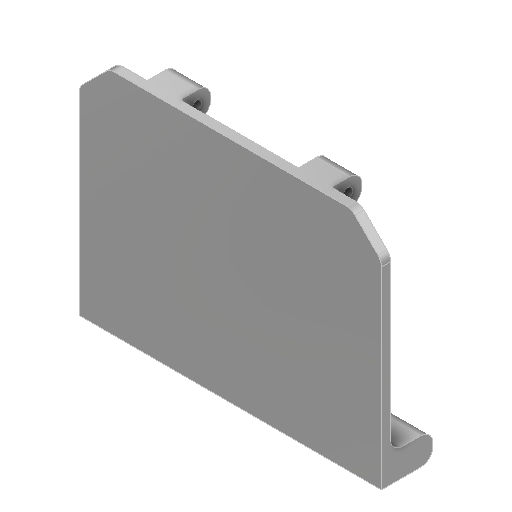
# Autodesk Inventor part: 3DP_PLA_Stand_Leg
Saved by Autodesk Inventor 2026.1 (Build 301233000, 233)
## iProperties
Created: 2024-09-01
Part Number: 3DP_PLA_Stand_Leg
Material: Generic
Document SubType Name: Modeling
Designer: User
Density: 1 g/cm^3
Appearance: Rubber - Black - Version 1.1
Author: User
Autodesk Inventor part; units mm, degrees
ref_plane "YZ Plane" through (0, 0, 0) normal (1, 0, 0) x (0, 1, 0)
ref_plane "XZ Plane" through (0, 0, 0) normal (0, 1, 0) x (-1, 0, 0)
ref_plane "XY Plane" through (0, 0, 0) normal (0, 0, 1) x (1, 0, 0)
sketch "Sketch1" plane through (0, 0, 0) normal (0, 0, 1) x (1, 0, 0)
  line L0 (-30.5, 4.5) -> (-19.5, 4.5)
  line L1 (-19.5, 4.5) -> (-19.5, -4.5)
  line L2 (-19.5, -4.5) -> (-30.5, -4.5)
  line L3 (-30.5, -4.5) -> (-30.5, 4.5)
  line L4 (19.5, 4.5) -> (30.5, 4.5)
  line L5 (30.5, 4.5) -> (30.5, -4.5)
  line L6 (30.5, -4.5) -> (19.5, -4.5)
  line L7 (19.5, -4.5) -> (19.5, 4.5)
  line L8 (-50, 4.5) -> (50, 4.5)
  line L9 (50, 4.5) -> (50, -71)
  line L10 (50, -71) -> (-50, -71)
  line L11 (-50, -71) -> (-50, 4.5)
  point P0 (0, 0)
  dimension "d0" = 11
  dimension "d1" = 9
  dimension "d2" = 19.5
  dimension "d3" = 4.5
  dimension "d4" = 11
  dimension "d5" = 19.5
  dimension "d6" = 9
  dimension "d7" = 100
  dimension "d8" = 50
  dimension "d9" = 4.5
  dimension "d10" = 71
  constraints: 24 end point, 6 parallel, 3 horizontal, 3 perpendicular
  measures "d0" distance of L1.end L2.end
  measures "d1" distance of L0.end L1.end
  measures "d2" distance from line of point (0, 0) L1
  measures "d3" distance from line of point (0, 0) L0
  measures "d4" distance of L4.start L4.end
  measures "d5" distance from line of point (0, 0) L7
  measures "d6" distance of L4.end L5.end
  measures "d7" distance between parallel lines of L9 L11
  measures "d8" distance from line of point (0, 0) L11
  measures "d9" distance from line of point (0, 0) L8
  measures "d10" distance from line of L10 point (0, 0)
extrude "Extrusion1" add sketch "Sketch1" along normal blind 3
extrude "Extrusion2" add sketch "Sketch1" against normal blind 10 contours L0 L1 L2 L3 | L4 L5 L6 L7
sketch "Sketch2" plane through (30.5, -4.5, 0) normal (1, 0, 0) x (0, 0, -1)
  line L0 (0, 0) -> (0, 9) projected
  line L1 (0, 0) -> (10, 0) projected
  line L2 (10, 9) -> (10, 0) projected
  line L3 (0, 9) -> (10, 9) projected
  point P0 (0, 4.5)
  point P1 (5.5, 4.5)
  dimension "d15" = 4.5
  dimension "d16" = 4.5
  measures "d15" distance from line of L3 point (5.5, 4.5)
  measures "d16" distance from line of L2 point (5.5, 4.5)
hole "Hole1" at (30.5, 0, -5.5) direction (-1, 0, 0) diameter 3.1 end through all
fillet "Fillet1" radius 4 6 edges at (25, 4.5, -10) (25, -4.5, -10) (-25, -4.5, -10) (-25, 4.5, -10) (-25, -4.5, 0) (25, -4.5, 0)
chamfer "Chamfer1" distance 10 angle 45 2 edges at (50, 4.5, 1.5) (-50, 4.5, 1.5)
sketch "Sketch3" plane through (0, 0, 0) normal (0, 0, -1) x (-1, 0, 0)
  line L0 (40, 4.5) -> (50, -5.5) projected
  line L1 (30.5, 4.5) -> (40, 4.5) projected
  line L2 (30.5, 4.5) -> (30.5, -8.5) projected
  line L3 (19.5, -8.5) -> (30.5, -8.5) projected
  line L4 (19.5, -8.5) -> (19.5, 4.5) projected
  line L5 (-19.5, 4.5) -> (19.5, 4.5) projected
  line L6 (-19.5, 4.5) -> (-19.5, -8.5) projected
  line L7 (-30.5, -8.5) -> (-19.5, -8.5) projected
  line L8 (-30.5, -8.5) -> (-30.5, 4.5) projected
  line L9 (-40, 4.5) -> (-30.5, 4.5) projected
  line L10 (-50, -5.5) -> (-40, 4.5) projected
  line L11 (-50, -71) -> (-50, -5.5) projected
  line L12 (50, -71) -> (-50, -71) projected
  line L13 (50, -5.5) -> (50, -71) projected
  line L14 (-50, -62) -> (50, -62)
  point P0 (0, 0)
  dimension "d28" = 9
  constraints: 2 end point, 2 point on line, 1 perpendicular
  measures "d28" distance between parallel lines of L12 L14
extrude "Extrusion3" add sketch "Sketch3" along normal blind 14 contours L13 L12 L11 L14
fillet "Fillet2" radius 4 3 edges at (0, -71, -14) (0, -62, -14) (0, -62, 0)
fillet "Fillet3" radius 4 4 edges at (-50, -5.5, 1.5) (-40, 4.5, 1.5) (40, 4.5, 1.5) (50, -5.5, 1.5)
equation "\"d3\" = 0.5 * d1"
equation "\"d4\" = d0"
equation "\"d5\" = d2"
equation "\"d8\" = 0.5 * d7"
equation "\"d16\" = d15"
body "Solid1"
